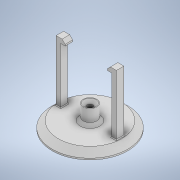
# Autodesk Inventor part: supportPoint2
Saved by Autodesk Inventor 2020.4 (Build 244396000, 396)
## iProperties
Created: 2022-03-09
Part Number: supportPoint2
Material: Generic
Document SubType Name: Modeling
Designer: Phabryan
Density: 1 g/cm^3
Appearance: Default
Author: Phabryan
Autodesk Inventor part; units mm, degrees
ref_plane "YZ Plane" through (0, 0, 0) normal (1, 0, 0) x (0, 1, 0)
ref_plane "XZ Plane" through (0, 0, 0) normal (0, 1, 0) x (-1, 0, 0)
ref_plane "XY Plane" through (0, 0, 0) normal (0, 0, 1) x (1, 0, 0)
sketch "Sketch1" plane through (0, 0, 0) normal (0, 1, 0) x (-1, 0, 0)
  circle A0 centre (0, 0) radius 25
  dimension "d0" = 50
  constraints: 1 centre point, 1 coincident
  measures "d0" diameter of A0
extrude "Extrusion1" add sketch "Sketch1" along normal blind 5
chamfer "Chamfer1" distance 4 angle 45 1 edges at (25, 5, 0)
sketch "Sketch2" plane through (0, 5, 0) normal (0, 1, 0) x (1, 0, 0)
  circle A0 centre (0, 0) radius 2
  circle A1 centre (0, 0) radius 4.5
  dimension "d6" = 4
  dimension "d7" = 9
  constraints: 2 centre point, 2 coincident
  measures "d6" diameter of A0
  measures "d7" diameter of A1
extrude "Extrusion2" add sketch "Sketch2" along normal blind 10
chamfer "Chamfer2" distance 2 angle 45 1 edges at (-4.5, 5, 0)
chamfer "Chamfer3" distance 2 angle 45 1 edges at (-2, 15, 0)
sketch "Sketch3" plane through (0, 5, 0) normal (0, 1, 0) x (1, 0, 0)
  line L0 (17, 2.5) -> (20, 2.5)
  line L1 (20, 2.5) -> (20, -2.5)
  line L2 (20, -2.5) -> (17, -2.5)
  line L3 (17, -2.5) -> (17, 2.5)
  point P0 (0, 0)
  dimension "d16" = 3
  dimension "d17" = 5
  dimension "d29" = 17
  constraints: 8 end point, 2 parallel, 1 horizontal, 1 perpendicular
  measures "d16" distance of L1.end L2.end
  measures "d17" distance of L0.end L1.end
  measures "d29" distance from line of point (0, 0) L3
extrude "Extrusion3" add sketch "Sketch3" along normal blind 40
sketch "Sketch4" plane through (17, 5, -2.5) normal (-1, 0, 0) x (0, 0, 1)
  line L0 (5, 40) -> (0, 40) projected
  line L1 (5, 0) -> (5, 40) projected
  line L2 (0, 40) -> (5, 40)
  line L3 (5, 40) -> (5, 37)
  line L4 (5, 37) -> (0, 37)
  line L5 (0, 37) -> (0, 40)
  point P0 (2.5, -5)
  dimension "d20" = 3
  constraints: 8 end point, 2 parallel, 1 horizontal, 1 perpendicular, 1 point on line
  measures "d20" distance of L2.end L3.end
extrude "Extrusion4" add sketch "Sketch4" along normal blind 3
chamfer "Chamfer4" distance 2 angle 45 1 edges at (14, 45, 0)
mirror "Mirror1" about plane through (0, 0, 0) normal (1, 0, 0) of "Extrusion3", "Chamfer4", "Extrusion4"
chamfer "Chamfer6" distance 0.5 angle 45 8 edges at (20, 5, 0) (18.5, 5, 2.5) (18.5, 5, -2.5) (17, 5, 0) (-17, 5, 0) (-18.5, 5, 2.5) (-20, 5, 0) (-17, 23.5, -2.5)
body "Solid1"
